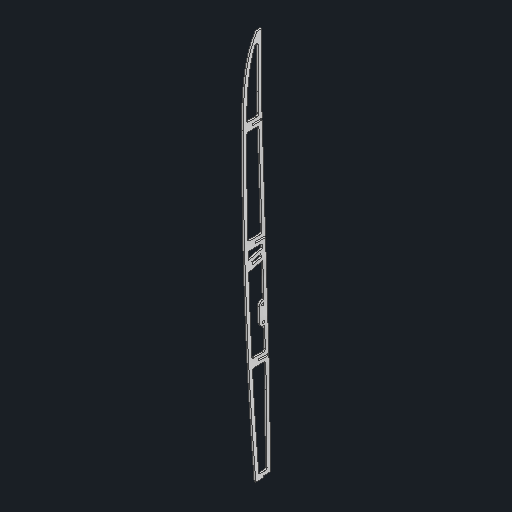
# Autodesk Inventor part: stringer_cowl
Saved by Autodesk Inventor 2023 (Build 270158030, 158C)
## iProperties
Created: 2022-03-23
Part Number: stringer_cowl
Material: Generic
Document SubType Name: Modeling
Designer: kardo
Density: 1 g/cm^3
Appearance: Default
Author: kardo
Autodesk Inventor part; units mm, degrees
ref_plane "YZ Plane" through (0, 0, 0) normal (1, 0, 0) x (0, 1, 0)
ref_plane "XZ Plane" through (0, 0, 0) normal (0, 1, 0) x (-1, 0, 0)
ref_plane "XY Plane" through (0, 0, 0) normal (0, 0, 1) x (1, 0, 0)
derived "parameters_frame.ipt"
derived "surface_body.ipt"
sketch "sk_rail_top_cowl" plane through (54.6, 0, 0) normal (1, 0, 0) x (0, 1, 0)
  spline S0 degree 2 poles (-363, 39.712) (-181.6483, 54.394) (0, 54.4) knots 0 0 0 1 1 1
  spline S1 degree 3 poles (0, 54.4) (52.14, 54.4) (75.84, 49.3408) (94.8, 37.536) knots 1 1 1 1 2 2 2 2
  point P0 (0, 0)
sketch "sk_rail_bottom_standoff" plane through (34.32, 0, 0) normal (1, 0, 0) x (0, 1, 0)
  line L0 (-363, 18.496) -> (-275.8801, 19.4795)
  arc A0 (-275.8801, 19.4795) -> (-254.1001, 19.9549) centre (-287.5515, 1053.3708) ccw
  line L1 (30.81, 28.832) -> (94.8, 28.832)
  arc A1 (30.81, 28.832) -> (9.48, 28.4869) centre (30.81, -630.4631) ccw
  line L2 (-254.1001, 19.9549) -> (9.48, 28.4869)
  line L3 (-483, 0) -> (357, 0) construction
  line L4 (9.48, 28.4869) -> (9.48, 0) construction
  line L5 (-254.1001, 19.9549) -> (-254.1001, 0) construction
  point P0 (0, 0)
  point P1 (-254.1001, 19.7253)
  point P2 (9.48, 28.832)
ref_plane "plane_middle" through (0, 0, 0) normal (0, 1, 0) x (-1, 0, 0)
ref_plane "plane_rear" through (0, -363, 0) normal (0, 1, 0) x (-1, 0, 0)
ref_plane "plane_cowl_right" through (54.6, 0, 0) normal (1, 0, 0) x (0, 1, 0)
ref_plane "plane_nose" through (0, 94.8, 0) normal (0, 1, 0) x (-1, 0, 0)
ref_plane "plane_tail_1" through (0, -120.9999, 0) normal (0, 1, 0) x (-1, 0, 0)
ref_plane "plane_tail_2" through (0, -242.0001, 0) normal (0, 1, 0) x (-1, 0, 0)
derived "stencil_frame.ipt"
sketch "sk_cowl_joint_locations" plane through (54.6, 0, 0) normal (1, 0, 0) x (0, 1, 0)
  line L0 (-363, 18.496) -> (-275.8801, 19.4795) construction
  arc A0 (-275.8801, 19.4795) -> (-254.1001, 19.9549) centre (-287.5515, 1053.3708) ccw construction
  line L1 (-254.1001, 19.9549) -> (9.48, 28.4869) construction
  arc A1 (30.81, 28.832) -> (9.48, 28.4869) centre (30.81, -630.4631) ccw construction
  line L2 (30.81, 28.832) -> (94.8, 28.832) construction
  line L3 (94.8, 30.032) -> (30.81, 30.032) construction
  arc A2 (30.81, 30.032) -> (9.4412, 29.6862) centre (30.81, -630.4631) ccw construction
  line L4 (9.4412, 29.6862) -> (-254.1389, 21.1542) construction
  arc A3 (-275.8936, 20.6794) -> (-254.1389, 21.1542) centre (-287.5515, 1053.3708) ccw construction
  line L5 (-275.8936, 20.6794) -> (-363, 19.6961) construction
  line L6 (-242.0001, 1541.8302) -> (-242.0001, -1877.3857) construction
  line L7 (-120.9999, 1541.8302) -> (-120.9999, -1877.3857) construction
  line L8 (-363, 1541.8302) -> (-363, -1877.3857) construction
  line L9 (0, 1541.8302) -> (0, -1877.3857) construction
  line L10 (-242.0001, 45.0688) -> (-242.0001, 21.5472) construction
  line L11 (-120.9999, 49.9661) -> (-120.9999, 25.4639) construction
  line L12 (-363, 19.6961) -> (-363, 19.6961)
  line L13 (-363, 19.6961) -> (-363, 36.9211) construction
  line L14 (-513.5712, 1550.2518) -> (344.0815, -1889.6051) construction
  line L15 (-362.7741, 36.9211) -> (-363, 39.712) construction
  spline S0 degree 2 poles (-363, 39.712) (-181.6483, 54.394) (0, 54.4) knots 0 0 0 1 1 1
  spline S1 degree 3 poles (0, 54.4) (52.14, 54.4) (75.84, 49.3408) (94.8, 37.536) knots 1 1 1 1 2 2 2 2
  line L16 (0, 51.6) -> (0, 29.3806) construction
  spline S2 degree 3 poles (93.3201, 35.1591) (91.7887, 36.1125) (88.6673, 37.9255) (84.5441, 39.9679) (80.1975, 41.8496) (76.5188, 43.2287) (71.6118, 44.7991) (67.4172, 45.9339) (61.7832, 47.203) (56.9422, 48.0997) (50.4217, 49.0741) (44.8094, 49.7373) (37.2484, 50.4231) (30.743, 50.8582) (21.9903, 51.263) (12.5916, 51.53) (4.3299, 51.6) (0, 51.6) knots 1 1 1 1 1.083333 1.166667 1.208333 1.291667 1.333333 1.416667 1.458333 1.541667 1.583333 1.666667 1.708333 1.791667 1.833333 1.916667 2 2 2 2
  spline S3 degree 3 poles (0, 51.6) (-20.1706, 51.5993) (-55.4643, 51.3605) (-95.7903, 50.6123) (-126.0307, 49.8474) (-146.1889, 49.2356) (-171.3841, 48.3435) (-191.5382, 47.528) (-216.7283, 46.3813) (-236.8783, 45.3621) (-262.0632, 43.9608) (-282.2091, 42.7379) (-307.3889, 41.082) (-332.5661, 39.2987) (-352.7052, 37.7363) (-362.7741, 36.9211) knots 0 0 0 0 0.166667 0.291667 0.333333 0.416667 0.458333 0.541667 0.583333 0.666666 0.708333 0.791666 0.833333 0.916666 1 1 1 1
  line L17 (-142.5135, 45.4866) -> (-137.389, 24.9334) construction
  line L18 (-134.789, 31.0394) -> (-138.6702, 30.0717) construction
  line L19 (-137.3512, 41.316) -> (-141.2324, 40.3483) construction
  line L20 (-142.5135, 45.4866) -> (-138.6324, 46.4543) construction
  line L21 (-137.389, 24.9334) -> (-133.5079, 25.9011) construction
  line L22 (-138.6324, 46.4543) -> (-138.8117, 52.2515) construction
  point P0 (0, 0)
  point P1 (-363, 28.3086)
  point P2 (-242.0001, 33.308)
  point P3 (-120.9999, 37.715)
  point P4 (0, 40.4903)
  point P5 (-513.5712, 1550.2518)
  point P6 (344.0815, -1889.6051)
  point P7 (-85.2629, 50.788)
  point P8 (0, 40.4903)
sketch "sk_servo_joint" plane through (-54.6, 0, 0) normal (1, 0, 0) x (0, 1, 0)
  line L0 (-254.1001, 19.9549) -> (9.48, 28.4869) construction
  line L1 (-363, 1541.8302) -> (-363, -1877.3857) construction
  line L2 (0, 1541.8302) -> (0, -1877.3857) construction
  line L3 (-204.8018, 21.5506) -> (-205.0153, 28.1472) construction
  line L4 (-205.0153, 28.1472) -> (-187.0247, 28.7295) construction
  line L5 (-187.0247, 28.7295) -> (-186.8112, 22.133) construction
  line L6 (-96.0723, 31.6736) -> (-99.3076, 131.6213) construction
  line L7 (-99.3076, 131.6213) -> (-199.2553, 128.386) construction
  line L8 (-199.2553, 128.386) -> (-196.02, 28.4384) construction
  line L9 (-187.0247, 28.7295) -> (-96.0723, 31.6736) construction
  point P0 (0, 0)
  point P1 (-191.0082, 43.6084)
sketch "sk_base" plane through (54.6, 0, 0) normal (1, 0, 0) x (0, 1, 0)
  line L0 (-363, 18.496) -> (-275.8801, 19.4795) construction
  arc A0 (-275.8801, 19.4795) -> (-254.1001, 19.9549) centre (-287.5515, 1053.3708) ccw construction
  line L1 (-254.1001, 19.9549) -> (9.48, 28.4869) construction
  arc A1 (30.81, 28.832) -> (9.48, 28.4869) centre (30.81, -630.4631) ccw construction
  line L2 (30.81, 28.832) -> (94.8, 28.832) construction
  spline S0 degree 3 poles (0, 54.4) (52.14, 54.4) (75.84, 49.3408) (94.8, 37.536) knots 1 1 1 1 2 2 2 2 construction
  spline S1 degree 2 poles (-363, 39.712) (-181.6483, 54.394) (0, 54.4) knots 0 0 0 1 1 1 construction
  line L3 (-363, 1390.1376) -> (-363, -967.2299) projected
  line L4 (94.8, 1390.1376) -> (94.8, -967.2299) construction
  line L5 (92.8, 30.032) -> (30.81, 30.032)
  arc A2 (30.81, 30.032) -> (9.4412, 29.6862) centre (30.81, -630.4631) ccw
  line L6 (9.4412, 29.6862) -> (-254.1389, 21.1542)
  arc A3 (-275.8936, 20.6794) -> (-254.1389, 21.1542) centre (-287.5515, 1053.3708) ccw
  line L7 (-275.8936, 20.6794) -> (-363.0135, 19.6959)
  line L8 (92.8, 35.4804) -> (92.8, 30.032)
  line L9 (-363, 39.712) -> (-362.7741, 36.9211) construction
  line L10 (-362.7741, 36.9211) -> (-363, 36.9028)
  spline S2 degree 4 poles (-362.7741, 36.9211) (-272.2777, 44.2476) (-181.5848, 49.1482) (-90.7923, 51.597) (0.0001, 51.6) knots 0 0 0 0 0 1 1 1 1 1
  spline S3 degree 5 poles (0, 51.6) (8.6623, 51.5996) (17.3257, 51.4847) (25.9841, 51.2081) (40.6061, 50.3871) (55.124, 48.5073) (61.0167, 47.5152) (71.2014, 45.2301) (80.9998, 41.6697) (85.0808, 39.882) (89.0143, 37.8005) (92.8, 35.4803) knots 0 0 0 0 0 0 0.45419 0.45419 0.45419 0.76719 0.76719 0.76719 1 1 1 1 1 1
  point P0 (0, 0)
  point P1 (-363, 19.6961)
  dimension "d3" = 2.8
  dimension "d2" = 1.2
  dimension "d4" = 2
  constraints: 12 end point, 4 point on circle, 2 centre point, 1 parallel, 1 perpendicular, 1 point on line, 12 other
  measures "d2" distance between parallel lines of L1 L6
  measures "d4" distance between parallel lines of L4 L8
extrude "thicken" add sketch "sk_base" along normal blind 2
sketch "sk_cut_weight" plane through (54.6, 0, 0) normal (1, 0, 0) x (0, 1, 0)
  spline S0 degree 3 poles (-362.7741, 36.9211) (-352.7052, 37.7363) (-332.5661, 39.2987) (-307.3889, 41.082) (-282.2091, 42.7379) (-262.0632, 43.9608) (-236.8782, 45.3622) (-216.7282, 46.3813) (-191.5382, 47.528) (-171.3841, 48.3435) (-146.1889, 49.2356) (-126.0307, 49.8474) (-95.7902, 50.6123) (-55.4642, 51.3605) (-20.1705, 51.5993) (0, 51.6) knots 0 0 0 0 0.083333 0.166667 0.208333 0.291667 0.333333 0.416667 0.458333 0.541667 0.583333 0.666667 0.708333 0.833333 1 1 1 1 construction
  line L0 (-275.8936, 20.6794) -> (-363.0135, 19.6959) construction
  line L1 (92.8, 35.4804) -> (92.8, 30.032) construction
  line L2 (-120.9999, 1390.1376) -> (-120.9999, -967.2299) construction
  line L3 (-242.0001, 1390.1376) -> (-242.0001, -967.2299) construction
  line L4 (-363, 1390.1376) -> (-363, -967.2299) construction
  line L5 (0, 1390.1376) -> (0, -967.2299) construction
  line L6 (9.4412, 29.6862) -> (-254.1389, 21.1542) construction
  arc A0 (-275.8936, 20.6794) -> (-254.1389, 21.1542) centre (-287.5515, 1053.3708) ccw construction
  line L7 (92.8, 30.032) -> (30.81, 30.032) construction
  arc A1 (30.81, 30.032) -> (9.4412, 29.6862) centre (30.81, -630.4631) ccw construction
  spline S1 degree 3 poles (0, 51.6) (4.2892, 51.6) (12.4768, 51.5313) (21.7997, 51.2693) (30.4878, 50.8723) (36.9499, 50.4454) (44.4658, 49.7727) (50.0487, 49.1222) (56.5394, 48.1665) (61.3615, 47.2871) (66.9766, 46.0423) (71.1592, 44.9294) (76.0533, 43.3895) (79.7229, 42.0373) (84.0576, 40.1926) (88.168, 38.1907) (91.2763, 36.4143) (92.8, 35.4804) knots 1 1 1 1 1.082549 1.165098 1.206372 1.288921 1.330196 1.412745 1.454019 1.536568 1.577842 1.660391 1.701666 1.784215 1.825489 1.908038 1.990587 1.990587 1.990587 1.990587 construction
  line L8 (-361, 19.6959) -> (-361, 51.6) construction
  line L9 (-240.0001, 51.6) -> (-240.0001, 19.6959) construction
  line L10 (-118.9999, 51.6) -> (-118.9999, 19.6959) construction
  line L11 (2, 51.6) -> (2, 19.6959) construction
  line L12 (-357, 33.3722) -> (-357, 23.7641)
  line L13 (-246.0001, 25.4198) -> (-246.0001, 40.8451)
  line L14 (-236.0001, 41.3831) -> (-236.0001, 25.7435)
  line L15 (-114.9999, 46.1227) -> (-114.9999, 29.6602)
  line L16 (-4, 33.2532) -> (-4, 47.5981)
  line L17 (6, 47.5764) -> (6, 33.5769)
  line L18 (87.3291, 34.032) -> (30.81, 34.032)
  arc A2 (30.81, 34.032) -> (9.3118, 33.6841) centre (30.81, -630.4631) ccw
  line L19 (9.3118, 33.6841) -> (-254.2683, 25.1521)
  arc A3 (-275.9388, 24.6791) -> (-254.2683, 25.1521) centre (-287.5515, 1053.3708) ccw
  line L20 (-275.9388, 24.6791) -> (-363.0587, 23.6957)
  line L21 (-124.9999, 45.8548) -> (-124.9999, 29.3365)
  spline S2 degree 4 poles (-362.4513, 32.9342) (-272.0355, 40.2541) (-181.4232, 45.1503) (-90.7115, 47.597) (0.0002, 47.6) knots 0 0 0 0 0 1 1 1 1 1
  spline S3 degree 5 poles (0, 47.6) (8.517, 47.5996) (17.035, 47.488) (25.5483, 47.2193) (39.8442, 46.4285) (54.0417, 44.6201) (59.7578, 43.6753) (68.8981, 41.6667) (77.7241, 38.6026) (81.0157, 37.2651) (84.2204, 35.7361) (87.3291, 34.032) knots 0 0 0 0 0 0 0.477132 0.477132 0.477132 0.801404 0.801404 0.801404 1 1 1 1 1 1
  point P0 (0, 0)
  dimension "d25" = 4
  dimension "d18" = 2
  dimension "d19" = 2
  dimension "d20" = 2
  dimension "d21" = 2
  dimension "d22" = 4
  dimension "d23" = 4
  dimension "d26" = 4
  dimension "d27" = 4
  dimension "d28" = 4
  dimension "d29" = 4
  dimension "d30" = 4
  constraints: 28 end point, 12 parallel, 8 horizontal alignment, 7 point on line, 4 point on circle, 2 centre point, 17 other
  measures "d18" distance between parallel lines of L3 L9
  measures "d19" distance between parallel lines of L10 L2
  measures "d20" distance between parallel lines of L11 L5
  measures "d21" distance between parallel lines of L8 L4
  measures "d22" distance between parallel lines of L8 L12
  measures "d23" distance between parallel lines of L13 L3
  measures "d26" distance between parallel lines of L9 L14
  measures "d27" distance between parallel lines of L10 L15
  measures "d28" distance between parallel lines of L16 L5
  measures "d29" distance between parallel lines of L11 L17
  measures "d30" distance between parallel lines of L21 L2
extrude "cut_weight" cut sketch "sk_cut_weight" along normal through all both and the other way through all contours S2 L13 L19 A3 L20 L12 | S2 L21 L19 L14 | S2 L16 L19 L15 | L17 S3 L18 A2 L19
fillet "rounding" radius 2 15 edges at (55.6, -246.0001, 25.4198) (55.6, -124.9999, 29.3365) (55.6, -4, 33.2532) (55.6, 87.3291, 34.032) (55.6, 6, 33.5769) (55.6, -114.9999, 29.6602) (55.6, -236.0001, 25.7435) (55.6, -357, 23.7641) (55.6, -357, 33.3722) (55.6, -236.0001, 41.3831) (55.6, -114.9999, 46.1227) (55.6, 6, 47.5764) (55.6, -4, 47.5981) (55.6, -124.9999, 45.8548) (55.6, -246.0001, 40.8451)
sketch "sk_joint_motor_mount" plane through (54.6, 0, 0) normal (1, 0, 0) x (0, 1, 0)
  spline S0 degree 3 poles (-362.7741, 36.9211) (-352.7052, 37.7363) (-332.5661, 39.2987) (-307.3889, 41.082) (-282.2091, 42.7379) (-262.0632, 43.9608) (-236.8782, 45.3622) (-216.7282, 46.3813) (-191.5382, 47.528) (-171.3841, 48.3435) (-146.1889, 49.2356) (-126.0307, 49.8474) (-95.7902, 50.6123) (-55.4642, 51.3605) (-20.1705, 51.5993) (0, 51.6) knots 0 0 0 0 0.083333 0.166667 0.208333 0.291667 0.333333 0.416667 0.458333 0.541667 0.583333 0.666667 0.708333 0.833333 1 1 1 1 projected
  line L0 (9.4412, 29.6862) -> (-254.1389, 21.1542) projected
  line L1 (-137.3512, 41.316) -> (-134.789, 31.0394) construction
  line L2 (-137.3512, 41.316) -> (-141.2324, 40.3483) construction
  line L3 (-141.2324, 40.3483) -> (-138.6702, 30.0717) construction
  line L4 (-138.6702, 30.0717) -> (-134.789, 31.0394) construction
  line L5 (-147.5546, 49.171) -> (-141.4785, 24.801)
  line L6 (-135.2837, 49.558) -> (-129.2101, 25.1981)
  point P0 (0, 0)
  dimension "d33" = 4
  dimension "d34" = 4
  dimension "d35" = 4
  constraints: 12 end point, 3 parallel, 2 coincident, 2 perpendicular, 2 point on line, 2 other
  measures "d33" distance between parallel lines of L1 L3
  measures "d34" distance between parallel lines of L3 L5
  measures "d35" distance between parallel lines of L1 L6
extrude "joint_motor_mount" add sketch "sk_joint_motor_mount" along normal blind 2
sketch "sk_joint_servo" plane through (54.6, 0, 0) normal (1, 0, 0) x (0, 1, 0)
  line L0 (9.4412, 29.6862) -> (-254.1389, 21.1542) projected
  line L1 (-181.6358, 23.5011) -> (-182.9143, 29.5923)
  arc A0 (-182.9143, 29.5923) -> (-187.1606, 32.9273) centre (-187.0247, 28.7295) ccw
  line L2 (-187.1606, 32.9273) -> (-205.1512, 32.345)
  arc A1 (-205.1512, 32.345) -> (-209.1729, 28.7423) centre (-205.0153, 28.1472) ccw
  line L3 (-209.1729, 28.7423) -> (-210.0548, 22.5812)
  point P0 (0, 0)
  dimension "d39" = 80
  dimension "d40" = 80
  dimension "d41" = 4.2
  constraints: 6 end point, 4 point on circle, 4 tangent, 2 centre point, 2 coincident, 2 point on line, 1 equal radius
  measures "d39" angle of L1 L0
  measures "d40" angle of L0 L3
  measures "d41" radius of A0
extrude "joint_servo" add sketch "sk_joint_servo" along normal blind 2
hole "drill_joint_servo" at (54.6, -205.0153, 28.1472) at (54.6, -187.0247, 28.7295) direction (1, 0, 0) diameter 3 end through all
sketch "sk_cowl_joint_cuts" plane through (54.6, 0, 0) normal (1, 0, 0) x (0, 1, 0)
  line L0 (-242.0001, 1390.1376) -> (-242.0001, -967.2299) projected
  line L1 (-120.9999, 1390.1376) -> (-120.9999, -967.2299) projected
  line L2 (0, 1390.1376) -> (0, -967.2299) projected
  line L3 (-363, 1390.1376) -> (-363, -967.2299) projected
  line L4 (-120.9999, -12.285) -> (-118.9999, -12.285)
  line L5 (-118.9999, -12.285) -> (-118.9999, 37.715)
  line L6 (-118.9999, 37.715) -> (-120.9999, 37.715)
  line L7 (0, -9.5097) -> (2, -9.5097)
  line L8 (2, -9.5097) -> (2, 40.4903)
  line L9 (2, 40.4903) -> (0, 40.4903)
  line L10 (-242.0001, 33.308) -> (-240.0001, 33.308)
  line L11 (-240.0001, 33.308) -> (-240.0001, -16.692)
  line L12 (-240.0001, -16.692) -> (-242.0001, -16.692)
  line L13 (-363, 28.3086) -> (-361, 28.3086)
  line L14 (-361, 28.3086) -> (-361, -21.6914)
  line L15 (-361, -21.6914) -> (-363, -21.6914)
  line L16 (-134.789, 31.0394) -> (-137.3512, 41.316)
  line L17 (-137.3512, 41.316) -> (-141.2324, 40.3483)
  line L18 (-141.2324, 40.3483) -> (-138.6702, 30.0717)
  line L19 (-138.6702, 30.0717) -> (-134.789, 31.0394)
  point P0 (0, 0)
  dimension "d8" = 2
  dimension "d15" = 50
  dimension "d16" = 4
  constraints: 33 end point, 11 parallel, 10 perpendicular, 4 point on line
  measures "d8" distance of L8.end L9.end
  measures "d15" distance of L7.end L8.end
  measures "d16" distance of L16.end L17.end
extrude "cut_joints" cut sketch "sk_cowl_joint_cuts" along normal through all
equation "\"d3\" = cowl_liner_thickness + cowl_shell_thickness"
equation "\"d2\" = shell_thickness"
equation "\"d4\" = bulkhead_thickness"
equation "\"d5\" = bulkhead_thickness"
equation "\"d25\" = bulkhead_inset"
equation "\"d18\" = bulkhead_thickness"
equation "\"d19\" = bulkhead_thickness"
equation "\"d20\" = bulkhead_thickness"
equation "\"d21\" = bulkhead_thickness"
equation "\"d22\" = bulkhead_inset"
equation "\"d23\" = bulkhead_inset"
equation "\"d26\" = bulkhead_inset"
equation "\"d27\" = bulkhead_inset"
equation "\"d28\" = bulkhead_inset"
equation "\"d29\" = bulkhead_inset"
equation "\"d30\" = bulkhead_inset"
equation "\"d38\" = 0.5 * bulkhead_inset"
equation "\"d33\" = 2 * bulkhead_thickness"
equation "\"d34\" = bulkhead_inset"
equation "\"d35\" = bulkhead_inset"
equation "\"d36\" = bulkhead_thickness"
equation "\"d41\" = 1.4 * drill_servo_mount_diam"
equation "\"d42\" = bulkhead_thickness"
equation "\"d44\" = drill_servo_mount_diam"
equation "\"d8\" = bulkhead_thickness"
equation "\"d16\" = 2 * bulkhead_thickness"
equation "\"cowl_liner_thickness\" = 1.2"
equation "\"cowl_shell_thickness\" = 1.6"
equation "\"shell_thickness\" = 1.2"
equation "\"bulkhead_thickness\" = 2"
equation "\"bulkhead_inset\" = 4"
equation "\"drill_servo_mount_diam\" = 3"
body "Solid1"
